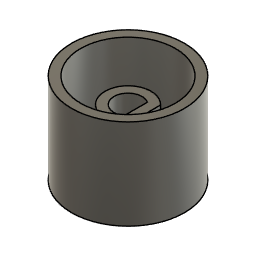
Knob (25mm) (Autodesk Fusion 360 design; units mm, degrees)
Autodesk Fusion 360 part; units mm, degrees
sketch "Outer" plane through (0, 0, 0) normal (0, 1, 0) x (1, 0, 0)
  circle A0 centre (0, 0) radius 12.5
  dimension "d1" = 25
  constraint coincident A0.centre origin
  measures "d1" diameter of A0
extrude "Outer Extrusion" add sketch "Outer" along normal blind 20
sketch "Inner" plane through (0, 20, 0) normal (0, 1, 0) x (-1, 0, 0)
  circle A0 centre (0, 0) radius 12.5
  circle A1 centre (0, 0) radius 10.5
  dimension "d4" = 21
  constraint coincident A0.centre A1.centre
  measures "d4" diameter of A1
extrude "Inner Extrusion" cut sketch "Inner" against normal blind 18 contours A1
sketch "Shaft" plane through (0, 2, 0) normal (0, 1, 0) x (-1, 0, 0)
  circle A0 centre (0, 0) radius 10.5
  line L0 (-1.7, 2.5923) -> (-1.7, -2.5923)
  arc A1 (-1.7, -2.5923) -> (-1.7, 2.5923) centre (0, 0) ccw
  arc A2 (-3.7, -3.51) -> (-3.7, 3.51) centre (0, 0) ccw
  line L1 (-3.7, 3.51) -> (-3.7, -3.51)
  dimension "d7" = 6.2
  dimension "d8" = 1.7
  dimension "d9" = 2
  constraint concentric A0 A1
  constraint vertical L0
  measures "d7" diameter of A1
  measures "d8" distance of A0.centre L0
extrude "Shaft Extrusion" add sketch "Shaft" along normal blind 12.5 contours A2 L1
equation "d4 = 25 mm - 2 mm - 2 mm"
equation "d5 = -( 20 mm - 2 mm )"
equation "d7 = 5.8 mm + 0.2 mm + 0.2 mm"
equation "d8 = ( 4.5 mm - 3 mm ) + 0.2 mm"
equation "d10 = 20 mm - 2 mm - 5.5 mm"
named bodies: "Body"
